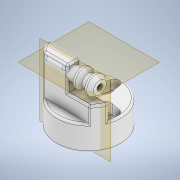
# Autodesk Inventor part: CablePlugBarbRA
Saved by Autodesk Inventor 2022 (Build 260153000, 153)
## iProperties
Created: 2021-10-25
Part Number: CablePlugBarbRA
Material: PC/ABS Plastic
Document SubType Name: Modeling
Designer: incep
Density: 0.357273 g/cm^3
Appearance: Smooth - White
Author: incep
Autodesk Inventor part; units mm, degrees
ref_plane "YZ Plane" through (0, 0, 0) normal (1, 0, 0) x (0, 1, 0)
ref_plane "XZ Plane" through (0, 0, 0) normal (0, 1, 0) x (-1, 0, 0)
ref_plane "XY Plane" through (0, 0, 0) normal (0, 0, 1) x (1, 0, 0)
sketch "Sketch1" plane through (0, 0, 0) normal (0, 1, 0) x (-1, 0, 0)
  circle A0 centre (0, 0) radius 16.5
  dimension "d0" = 33
  constraints: 1 centre point, 1 coincident
  measures "d0" diameter of A0
extrude "Extrusion1" add sketch "Sketch1" along normal blind 13
sketch "Sketch2" plane through (0, 0, 0) normal (0, -1, 0) x (1, 0, 0)
  line L0 (-8, 4.9075) -> (-3.75, 2.4537)
  line L1 (-3.75, 2.4537) -> (-3.75, -2.4537)
  line L2 (-3.75, -2.4537) -> (-8, -4.9075)
  line L3 (-8, -4.9075) -> (-12.25, -2.4537)
  line L4 (-12.25, -2.4537) -> (-12.25, 2.4537)
  line L5 (-12.25, 2.4537) -> (-8, 4.9075)
  line L6 (-4.9075, -8) -> (-2.4537, -3.75)
  line L7 (-2.4537, -3.75) -> (2.4537, -3.75)
  line L8 (2.4537, -3.75) -> (4.9075, -8)
  line L9 (4.9075, -8) -> (2.4537, -12.25)
  line L10 (2.4537, -12.25) -> (-2.4537, -12.25)
  line L11 (-2.4537, -12.25) -> (-4.9075, -8)
  line L12 (8, -4.9075) -> (3.75, -2.4537)
  line L13 (3.75, -2.4537) -> (3.75, 2.4537)
  line L14 (3.75, 2.4537) -> (8, 4.9075)
  line L15 (8, 4.9075) -> (12.25, 2.4537)
  line L16 (12.25, 2.4537) -> (12.25, -2.4537)
  line L17 (12.25, -2.4537) -> (8, -4.9075)
  circle A0 centre (-8, 0) radius 2.16
  circle A1 centre (0, -8) radius 2.16
  circle A2 centre (8, 0) radius 2.16
  circle A3 centre (-9.1924, -9.1924) radius 1.5
  line L18 (0, 0) -> (-9.1924, -9.1924) construction
  line L19 (0, 0) -> (-28.7343, 0) construction
  dimension "d7" = 8.5
  dimension "d8" = 8
  dimension "d9" = 180
  dimension "d10" = 4.32
  dimension "d11" = 180
  dimension "d16" = 3
  dimension "d17" = 45
  dimension "d18" = 13
  constraints: 40 end point, 4 centre point, 1 coincident, 1 horizontal, 1 horizontal alignment, 45 other
  measures "d7" distance between parallel lines of L5 L2
  measures "d8" distance of L18.start point (-8, 0)
  measures "d10" diameter of A0
  measures "d16" diameter of A3
  measures "d17" angle of L19 L18
  measures "d18" distance of L18.end point (0, 0)
extrude "Extrusion2" cut sketch "Sketch2" against normal blind 5 contours L0 L1 L2 L3 L4 L5 | L6 L7 L8 L9 L10 L11 | L12 L13 L14 L15 L16 L17 | A0 | A1 | A2
extrude "Extrusion3" cut sketch "Sketch2" against normal blind 8 contours A0 | A1 | A2
extrude "Extrusion4" cut sketch "Sketch2" against normal blind 0.5 contours A3
sketch "Sketch3" plane through (0, 13, 0) normal (0, 1, 0) x (1, 0, 0)
  circle A0 centre (-8, 0) radius 2.16 construction
  arc A1 (-8.7, -3.4293) -> (-8.7, 3.4293) centre (-8, 0) ccw
  line L0 (-8, 0) -> (-13, 0) construction
  arc A2 (-13.5, 2.4495) -> (-13.5, -2.4495) centre (-13, 0) ccw
  line L1 (-13.5, 2.4495) -> (-8.7, 3.4293)
  line L2 (-13.5, -2.4495) -> (-8.7, -3.4293)
  circle A3 centre (0, 8) radius 2.16 construction
  arc A4 (-3.4293, 8.7) -> (3.4293, 8.7) centre (0, 8) ccw
  line L3 (0, 8) -> (0, 13) construction
  arc A5 (2.4495, 13.5) -> (-2.4495, 13.5) centre (0, 13) ccw
  line L4 (2.4495, 13.5) -> (3.4293, 8.7)
  line L5 (-2.4495, 13.5) -> (-3.4293, 8.7)
  circle A6 centre (8, 0) radius 2.16 construction
  arc A7 (8.7, 3.4293) -> (8.7, -3.4293) centre (8, 0) ccw
  line L6 (8, 0) -> (13, 0) construction
  arc A8 (13.5, -2.4495) -> (13.5, 2.4495) centre (13, 0) ccw
  line L7 (13.5, -2.4495) -> (8.7, -3.4293)
  line L8 (13.5, 2.4495) -> (8.7, 3.4293)
  point P0 (0, 0)
  dimension "d21" = 8
  dimension "d22" = 4.32
  dimension "d23" = 7
  dimension "d24" = 5
  dimension "d25" = 5
  dimension "d28" = 180
  constraints: 18 end point, 12 point on circle, 9 centre point, 6 coincident, 4 tangent, 1 horizontal, 1 horizontal alignment, 29 other
  measures "d21" distance of point (0, 0) A0.centre
  measures "d22" diameter of A0
  measures "d23" diameter of A1
  measures "d24" distance of L0.start L0.end
  measures "d25" diameter of A2
extrude "Extrusion5" cut sketch "Sketch3" against normal blind 5
sketch "Sketch4" plane through (0, 13, 0) normal (0, 1, 0) x (1, 0, 0)
  line L0 (-15.7242, -5) -> (15.7242, -5)
  line L1 (11.8068, -11.526) -> (-11.8068, -11.526)
  arc A0 (-15.7242, -5) -> (-11.8068, -11.526) centre (0, 0) ccw
  arc A1 (11.8068, -11.526) -> (15.7242, -5) centre (0, 0) ccw
  dimension "d32" = 5
  dimension "d33" = 6.526
  dimension "d111" = 16.5
  dimension "d112" = 16.5
  constraints: 4 end point, 4 point on circle, 2 centre point, 1 coincident, 1 horizontal, 1 parallel
  measures "d32" distance from line of L0 point (0, 0)
  measures "d33" distance between parallel lines of L1 L0
  measures "d111" radius of A0
  measures "d112" radius of A1
extrude "Extrusion6" add sketch "Sketch4" along normal blind 20.525
sketch "Sketch11" plane through (15.7242, 13, 5) normal (0, 0, -1) x (-1, 0, 0)
  line L0 (0, 0) -> (0, 20.525) projected
  line L1 (0, 20.525) -> (15, 20.525)
  line L2 (15, 20.525) -> (15, 8)
  line L3 (15, 8) -> (0, 8)
  line L4 (0, 8) -> (0, 20.525)
  line L5 (32.2242, 0) -> (-0.7758, 0) projected
  point P0 (15.7242, -13)
  point P1 (31.4484, 0)
  point P2 (0, 8)
  dimension "d117" = 8
  dimension "d118" = 15
  constraints: 8 end point, 2 parallel, 1 horizontal, 1 perpendicular
  measures "d117" distance between parallel lines of L5 L3
  measures "d118" distance of L2.end L3.end
ref_plane "Work Plane2" through (-11.8068, 13, 8.263) normal (0, 0, 1) x (1, 0, 0)
extrude "Extrusion11" cut sketch "Sketch11" against normal blind 10
sketch "Sketch9" plane through (-11.8068, 13, 8.263) normal (0, 0, 1) x (1, 0, 0)
  line L0 (11.8068, 15.7625) -> (11.8068, 11) construction
  line L1 (11.8068, 11) -> (25.8068, 11) construction
  line L2 (25.8068, 11) -> (25.8068, 15.7625) construction
  line L3 (25.8068, 15.7625) -> (11.8068, 15.7625) construction
  line L4 (16.8068, 12.5) -> (16.8068, 11) construction
  line L5 (16.8068, 11) -> (19.8068, 11) construction
  line L6 (19.8068, 11) -> (19.8068, 12.5) construction
  line L7 (19.8068, 12.5) -> (16.8068, 12.5) construction
  line L8 (19.8068, 12.5) -> (19.8068, 11) construction
  line L9 (19.8068, 11) -> (22.8068, 11) construction
  line L10 (22.8068, 11) -> (22.8068, 12.5) construction
  line L11 (22.8068, 12.5) -> (19.8068, 12.5) construction
  line L12 (22.8068, 12.5) -> (22.8068, 11) construction
  line L13 (22.8068, 11) -> (25.8068, 11) construction
  line L14 (25.8068, 11) -> (25.8068, 12.5) construction
  line L15 (25.8068, 12.5) -> (22.8068, 12.5) construction
  line L16 (11.8068, 14.25) -> (25.8068, 14.25) construction
  line L17 (16.8068, 12.5) -> (11.8068, 12.5) construction
  line L18 (11.8068, 12.5) -> (16.8068, 12.5)
  line L19 (16.8068, 11) -> (17.8068, 11)
  line L20 (17.8068, 11) -> (19.8068, 12.5)
  line L21 (16.8068, 12.5) -> (16.8068, 11)
  line L22 (19.8068, 12.5) -> (22.8068, 12.5)
  line L23 (22.8068, 12.5) -> (22.8068, 11)
  line L24 (22.8068, 11) -> (23.8068, 11)
  line L25 (23.8068, 11) -> (25.8068, 12.5)
  line L26 (25.8068, 12.5) -> (25.8068, 14.25)
  line L27 (25.8068, 14.25) -> (11.8068, 14.25)
  line L28 (11.8068, 14.25) -> (11.8068, 12.5)
  line L29 (23.6137, 0) -> (0, 0) projected
  point P0 (11.8068, -13)
  dimension "d102" = 4.7625
  dimension "d103" = 1.5
  dimension "d104" = 3
  dimension "d105" = 5
  dimension "d106" = 1.75
  dimension "d107" = 1
  dimension "d108" = 1
  dimension "d109" = 11
  constraints: 58 end point, 8 parallel, 8 perpendicular, 8 point on line, 6 collinear, 1 vertical alignment
  measures "d102" distance of L1.end L2.end
  measures "d103" distance of L5.end L6.end
  measures "d104" distance of L4.end L5.end
  measures "d105" distance between parallel lines of L4 L0
  measures "d106" distance between parallel lines of L15 L16
  measures "d107" distance of L4.end L19.end
  measures "d108" distance of L12.end L24.end
  measures "d109" distance between parallel lines of L1 L29
revolve "Revolution2" add sketch "Sketch9" angle 360 about axis through (14, 28.7625, 8.263) along (-1, 0, 0)
sketch "Sketch12" plane through (0.7242, 21, 5) normal (1, 0, 0) x (0, 0, -1)
  line L0 (-6.526, -8) -> (-6.526, 12.525) projected
  line L1 (-6.526, 7.763) -> (0, 7.763) construction
  line L2 (0, -8) -> (0, 12.525) projected
  line L3 (21.5, -8) -> (0, -8) construction
  circle A0 centre (-3.263, 7.763) radius 1.5065
  point P0 (5, -21)
  dimension "d121" = 15.763
  dimension "d122" = 3.013
  constraints: 2 end point, 2 point on line, 1 centre point, 1 horizontal, 1 midpoint
  measures "d121" distance between parallel lines of L3 L1
  measures "d122" diameter of A0
ref_plane "Work Plane3" through (0.7242, 28.763, 8.263) normal (0, 1, 0) x (1, 0, 0)
sketch "Sketch13" plane through (0.7242, 28.763, 8.263) normal (0, 1, 0) x (1, 0, 0)
  line L0 (0, 3.263) -> (0, -3.263) projected
  line L1 (-16.4484, 3.263) -> (15, 3.263) projected
  line L2 (0, 0) -> (-11.1105, 0) construction
  line L3 (-11.1105, 0) -> (-14.5986, 3.263) construction
  line L4 (-14.5986, 3.263) -> (-15.5492, 5.977) construction
  spline S0 degree 3 poles (0, 0) (-11.1105, 0) (-14.5986, 3.263) (-15.5492, 5.977) knots 1 1 1 1 2 2 2 2
  point P0 (-0.7242, 8.263)
  constraints: 1 midpoint, 1 point on line, 3 other
sweep "Sweep2" cut profiles "Sketch12" path "Sketch13" path curves S0
sketch "Sketch14" plane through (15.7242, 13, 5) normal (0, 0, -1) x (-1, 0, 0)
  line L0 (17, 19.525) -> (27, 19.525)
  line L1 (27, 17.525) -> (17, 17.525)
  arc A0 (27, 17.525) -> (27, 19.525) centre (27, 18.525) ccw
  arc A1 (17, 19.525) -> (17, 17.525) centre (17, 18.525) ccw
  line L2 (15, 20.525) -> (15, 8) projected
  line L3 (15, 20.525) -> (31.4484, 20.525) projected
  line L4 (16, 18.525) -> (28, 18.525)
  point P0 (15.7242, -13)
  dimension "d127" = 2
  dimension "d128" = 10
  dimension "d129" = 2
  dimension "d130" = 2
  constraints: 6 end point, 6 point on circle, 4 tangent, 2 centre point, 1 horizontal, 1 parallel
  measures "d127" distance between parallel lines of L1 L0
  measures "d128" distance of L1.start L1.end
  measures "d129" distance from line of L2 A1.centre
  measures "d130" distance from line of L3 A1.centre
revolve "Revolution3" add sketch "Sketch14" angle 360 about axis through (-0.2758, 31.525, 5) along (-1, 0, 0) contours L0 A0 L4 A1
sketch "Sketch15" plane through (-11.8068, 13, 11.526) normal (0, 0, 1) x (1, 0, 0)
  line L0 (2.531, 19.525) -> (10.531, 19.525)
  line L1 (10.531, 17.525) -> (2.531, 17.525)
  arc A0 (10.531, 17.525) -> (10.531, 19.525) centre (10.531, 18.525) ccw
  arc A1 (2.531, 19.525) -> (2.531, 17.525) centre (2.531, 18.525) ccw
  line L2 (1.531, 18.525) -> (11.531, 18.525)
  line L3 (12.531, 8) -> (12.531, 20.525) projected
  line L4 (0, 20.525) -> (12.531, 20.525) projected
  point P0 (11.8068, -13)
  point P1 (15.7242, -13)
  dimension "d132" = 2
  dimension "d133" = 8
  dimension "d136" = 2
  dimension "d137" = 2
  constraints: 6 end point, 6 point on circle, 4 tangent, 2 centre point, 1 horizontal, 1 parallel
  measures "d132" distance between parallel lines of L1 L0
  measures "d133" distance of L1.start L1.end
  measures "d136" distance from line of L3 A0.centre
  measures "d137" distance from line of L4 A0.centre
revolve "Revolution4" add sketch "Sketch15" angle 360 about axis through (-10.2758, 31.525, 11.526) along (1, 0, 0) contours L0 A0 L2 A1
fillet "Fillet2" radius 1 17 edges at (14.147, 21, 8.492) (8.2242, 21, 5) (6.2655, 21, 11.526) (0.7242, 27.2625, 11.526) (0.7242, 27.2625, 5) (0.7242, 33.525, 8.263) (-5.5413, 33.525, 11.526) (-7.5, 33.525, 5) (-14.147, 33.525, 8.492) (-15.7242, 23.2625, 5) (-11.8068, 23.2625, 11.526) (0, 13, 16.5) (-16.3049, 13, 2.5299) (2.5299, 13, -16.3049) (11.8068, 17, 11.526) (15.7242, 17, 5) (16.5, 0, 0)
body "Solid1"
